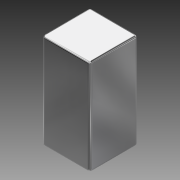
# Autodesk Inventor part: magnet1_4x1_4x1_2
Saved by Autodesk Inventor 2013 (Build 170138000, 138)
## iProperties
Created: 2013-01-21
Part Number: magnet1_4x1_4x1_2
Material: Nickel-Copper Alloy 400
Document SubType Name: Modeling
Designer: Nano
Density: 8.83 g/cm^3
Mass: 4.52181 g
Surface Area: 4.03225 cm^2
Volume: 0.512096 cm^3
Author: Nano
Autodesk Inventor part; units mm, degrees
ref_plane "YZ Plane" through (0, 0, 0) normal (1, 0, 0) x (0, 1, 0)
ref_plane "XZ Plane" through (0, 0, 0) normal (0, 1, 0) x (-1, 0, 0)
ref_plane "XY Plane" through (0, 0, 0) normal (0, 0, 1) x (1, 0, 0)
sketch "Sketch1" plane through (0, 0, 0) normal (0, 1, 0) x (-1, 0, 0)
  line L0 (-3.175, -3.175) -> (3.175, -3.175)
  line L1 (3.175, -3.175) -> (3.175, 3.175)
  line L2 (3.175, 3.175) -> (-3.175, 3.175)
  line L3 (-3.175, 3.175) -> (-3.175, -3.175)
  line L4 (-3.175, -3.175) -> (3.175, 3.175) construction
  line L5 (3.175, -3.175) -> (-3.175, 3.175) construction
  point P0 (0, 0)
  dimension "d0" = 6.35
  dimension "d1" = 6.35
  constraints: 12 end point, 2 midpoint, 2 parallel, 1 horizontal, 1 perpendicular
  measures "d0" distance of L2.end L1.end
  measures "d1" distance of L1.end L0.end
extrude "Extrusion1" add sketch "Sketch1" along normal blind 12.7
fillet "Fillet1" radius 0.3175 12 edges at (0, 12.7, 3.175) (3.175, 12.7, 0) (0, 12.7, -3.175) (-3.175, 12.7, 0) (-3.175, 6.35, 3.175) (3.175, 6.35, 3.175) (3.175, 6.35, -3.175) (-3.175, 6.35, -3.175) (0, 0, -3.175) (-3.175, 0, 0) (0, 0, 3.175) (3.175, 0, 0)
body "Solid1"
